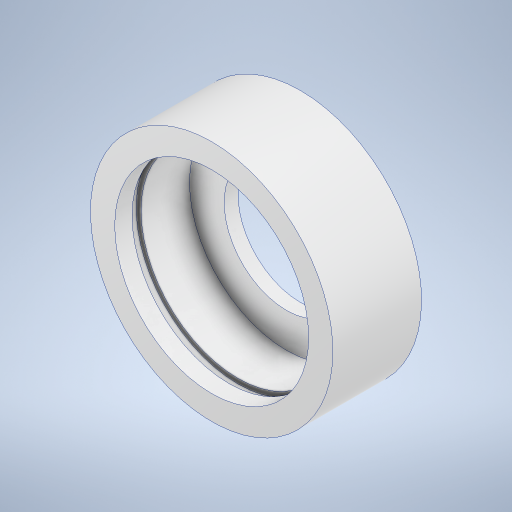
# Autodesk Inventor part: P401
Saved by Autodesk Inventor 2023 (Build 270158000, 158)
## iProperties
Created: 2022-08-29
Part Number: P401
Material: Aluminum 6061
Document SubType Name: Modeling
Designer: D.C. Eksteen
Density: 2.7 g/cm^3
Appearance: Aluminum - Flat
Author: D.C. Eksteen
Title: BEARING MOUNT
Autodesk Inventor part; units mm, degrees
ref_plane "YZ Plane" through (0, 0, 0) normal (1, 0, 0) x (0, 1, 0)
ref_plane "XZ Plane" through (0, 0, 0) normal (0, 1, 0) x (-1, 0, 0)
ref_plane "XY Plane" through (0, 0, 0) normal (0, 0, 1) x (1, 0, 0)
sketch "Sketch5" plane through (0, 0, 0) normal (1, 0, 0) x (0, 1, 0)
  line L0 (0, 0) -> (17.5, 0)
  line L1 (17.5, 0) -> (17.5, 12.8)
  line L2 (17.5, 12.8) -> (14, 12.8)
  line L3 (14, 12.8) -> (14, 10.3)
  line L4 (14, 10.3) -> (14.7, 10.3)
  line L5 (14.7, 10.3) -> (14.7, 9)
  line L6 (14.7, 9) -> (14, 9)
  line L7 (14, 9) -> (14, 2)
  line L8 (14, 2) -> (9, 2)
  line L9 (9, 2) -> (9, 0)
  line L10 (0, 0) -> (0, 12.8)
  dimension "d19" = 17.5
  dimension "d20" = 2.5
  dimension "d21" = 1.3
  dimension "d22" = 7
  dimension "d23" = 2
  dimension "d24" = 14.7
  dimension "d25" = 14
  dimension "d26" = 9
  constraints: 22 end point, 8 perpendicular, 3 point on line, 1 horizontal, 1 horizontal alignment, 1 vertical
  measures "d19" distance of L0.start L0.end
  measures "d20" distance of L2.end L3.end
  measures "d21" distance of L4.end L5.end
  measures "d22" distance of L6.end L7.end
  measures "d23" distance of L8.end L9.end
  measures "d24" distance from line of L0.start L5
  measures "d25" distance from line of L0.start L7
  measures "d26" distance from line of L0.start L9
revolve "Revolution1" add sketch "Sketch5" angle 360 about axis through (0, 0, 0) along (0, 0, 1)
body "Solid2"
